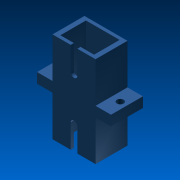
# Autodesk Inventor part: SC-adapter
Saved by Autodesk Inventor 2011 (Build 150239000, 239)
## iProperties
Created: 2010-06-01
Part Number: SC-adapter
Material: ABS Plastic
Document SubType Name: Modeling
Designer: Martins
Mass: 1.53166 g
Surface Area: 24.6742 cm^2
Volume: 1.44497 cm^3
Density: 1.06 g/cm^3
Author: Martins
Autodesk Inventor part; units mm, degrees
ref_plane "YZ Plane" through (0, 0, 0) normal (1, 0, 0) x (0, 1, 0)
ref_plane "XZ Plane" through (0, 0, 0) normal (0, 1, 0) x (-1, 0, 0)
ref_plane "XY Plane" through (0, 0, 0) normal (0, 0, 1) x (1, 0, 0)
sketch "Sketch1" plane through (0, 0, 0) normal (0, 0, 1) x (1, 0, 0)
  line L0 (-19.6117, 15.4854) -> (2.3883, 15.4854)
  line L1 (2.3883, 15.4854) -> (2.3883, 5.9854)
  line L2 (2.3883, 5.9854) -> (-19.6117, 5.9854)
  line L3 (-19.6117, 5.9854) -> (-19.6117, 15.4854)
  circle A0 centre (-17.6117, 10.7354) radius 1
  circle A1 centre (0.3883, 10.7354) radius 1
  point P0 (2.3883, 10.7354)
  dimension "d0" = 22
  dimension "d1" = 9.5
  dimension "d2" = 18
  dimension "d3" = 2
  dimension "d4" = 2
  constraints: 8 end point, 2 centre point, 2 horizontal alignment, 1 equal radius, 1 midpoint
  measures "d0" distance of L1.end L2.end
  measures "d1" distance of L2.end L0.start
  measures "d2" distance of A1.centre A0.centre
  measures "d3" distance from line of L3 A0.centre
  measures "d4" diameter of A1
extrude "Extrusion1" add sketch "Sketch1" along normal blind 3
sketch "Sketch2" plane through (0, 0, 3) normal (0, 0, 1) x (1, 0, 0)
  line L0 (-19.6117, 15.4854) -> (2.3883, 15.4854) projected
  line L1 (-19.6117, 5.9854) -> (-19.6117, 15.4854) projected
  line L2 (2.3883, 5.9854) -> (-19.6117, 5.9854) projected
  line L3 (-15.0117, 15.4854) -> (-2.2117, 15.4854)
  line L4 (-2.2117, 15.4854) -> (-2.2117, 5.9854)
  line L5 (-2.2117, 5.9854) -> (-15.0117, 5.9854)
  line L6 (-15.0117, 5.9854) -> (-15.0117, 15.4854)
  point P0 (0, 0)
  point P1 (-8.6117, 5.9854)
  point P2 (-8.6117, 5.9854)
  dimension "d7" = 12.8
  constraints: 8 end point, 2 collinear, 2 midpoint, 1 coincident, 1 parallel
  measures "d7" distance between parallel lines of L4 L6
extrude "Extrusion2" add sketch "Sketch2" along normal blind 12 contours L0 L4 L2 L6
sketch "Sketch3" plane through (0, 0, 0) normal (0, 0, -1) x (-1, 0, 0)
  line L0 (19.6117, 15.4854) -> (-2.3883, 15.4854) projected
  line L1 (-2.3883, 5.9854) -> (19.6117, 5.9854) projected
  line L2 (15.0117, 5.9854) -> (2.2117, 5.9854)
  line L3 (2.2117, 5.9854) -> (2.2117, 15.4854)
  line L4 (2.2117, 15.4854) -> (15.0117, 15.4854)
  line L5 (15.0117, 15.4854) -> (15.0117, 5.9854)
  point P0 (0, 0)
  point P1 (8.6117, 5.9854)
  point P2 (8.6117, 5.9854)
  dimension "d10" = 12.8
  constraints: 8 end point, 2 collinear, 2 midpoint, 1 coincident, 1 perpendicular
  measures "d10" distance between parallel lines of L3 L5
extrude "Extrusion3" add sketch "Sketch3" along normal blind 12
sketch "Sketch4" plane through (0, 0, -12) normal (0, 0, -1) x (-1, 0, 0)
  line L0 (2.2117, 5.9854) -> (2.2117, 15.4854) projected
  line L1 (15.0117, 5.9854) -> (2.2117, 5.9854) projected
  line L2 (13.6117, 6.9354) -> (3.6117, 6.9354)
  line L3 (3.6117, 6.9354) -> (3.6117, 14.5354)
  line L4 (3.6117, 14.5354) -> (13.6117, 14.5354)
  line L5 (13.6117, 14.5354) -> (13.6117, 6.9354)
  point P0 (0, 0)
  point P1 (8.6117, 5.9854)
  point P2 (8.6117, 6.9354)
  point P3 (3.6117, 10.7354)
  point P4 (2.2117, 10.7354)
  dimension "d13" = 10
  dimension "d14" = 7.6
  constraints: 8 end point, 4 midpoint, 3 parallel, 1 horizontal alignment, 1 perpendicular, 1 vertical alignment
  measures "d13" distance of L3.end L4.end
  measures "d14" distance of L2.end L3.end
extrude "Extrusion4" cut sketch "Sketch4" against normal blind 30
sketch "Sketch5" plane through (-19.6117, 5.9854, 0) normal (0, -1, 0) x (1, 0, 0)
  line L0 (17.4, 15) -> (4.6, 15) projected
  line L1 (4.6, 3) -> (4.6, 15) projected
  line L2 (4.6, 0) -> (4.6, -12) projected
  line L3 (4.6, -12) -> (17.4, -12) projected
  arc A0 (10, 8) -> (12, 8) centre (11, 8) ccw
  arc A1 (12, -5) -> (10, -5) centre (11, -5) ccw
  line L4 (10, 8) -> (10, 15)
  line L5 (12, 8) -> (12, 15)
  line L6 (10, -5) -> (10, -12)
  line L7 (12, -5) -> (12, -12)
  point P0 (19.6117, 0)
  point P1 (11, 15)
  dimension "d17" = 7
  dimension "d18" = 7
  dimension "d19" = 2
  constraints: 8 end point, 4 parallel, 4 point on circle, 4 point on line, 4 tangent, 2 centre point, 2 vertical alignment, 1 equal radius, 1 midpoint
  measures "d17" distance from line of L0 A0.centre
  measures "d18" distance from line of L3 A1.centre
  measures "d19" diameter of A0
extrude "Extrusion5" cut sketch "Sketch5" against normal blind 3
body "Solid1"
